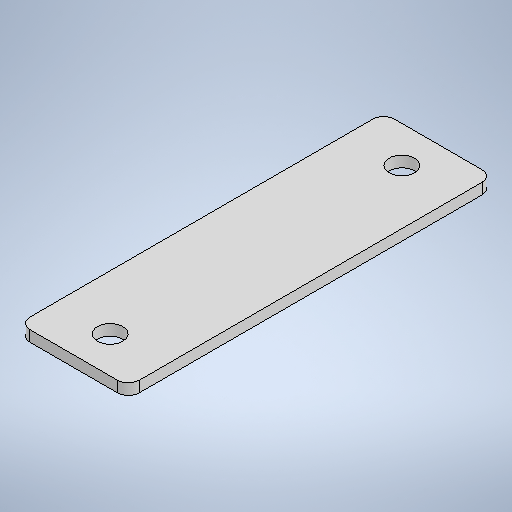
# Autodesk Inventor part: Part2
Saved by Autodesk Inventor 2025 (Build 290162010, 162A)
## iProperties
Created: 2025-11-03
Part Number: Part2
Material: Generic
Description: DIE16(5)|\ 90°|corrY -___°|X_____|bom___
Document SubType Name: Sheet Metal
Designer: admin
Stock Number: МОО 305 шпангоут борт
Mass: 186.989 g
Surface Area: 677.943 cm^2
Volume: 186.989 cm^3
Density: 1 g/cm^3
Sheet Metal Rule: Default
Sheet Metal Width: 0.000 mm
Sheet Metal Length: 0.000 mm
Sheet Metal Area: 0.000 mm^2
Appearance: Default
Author: admin
Autodesk Inventor part; units mm, degrees
ref_plane "YZ Plane" through (0, 0, 0) normal (1, 0, 0) x (0, 1, 0)
ref_plane "XZ Plane" through (0, 0, 0) normal (0, 1, 0) x (-1, 0, 0)
ref_plane "XY Plane" through (0, 0, 0) normal (0, 0, 1) x (1, 0, 0)
sketch "Sketch1" plane through (0, 0, 0) normal (0, 0, 1) x (1, 0, 0)
  line L0 (-30, -100) -> (30, -100)
  line L1 (30, -100) -> (30, 100)
  line L2 (30, 100) -> (-30, 100)
  line L3 (-30, 100) -> (-30, -100)
  line L4 (-30, -100) -> (30, 100) construction
  line L5 (30, -100) -> (-30, 100) construction
  circle A0 centre (0, 80) radius 7
  circle A1 centre (0, -80) radius 7
  line L6 (0, 100) -> (0, -100) construction
  line L7 (-30, 0) -> (30, 0) construction
  point P0 (0, 0)
  point P1 (0, 0)
  dimension "d154" = 60
  dimension "d155" = 200
  dimension "d157" = 20
  dimension "d159" = 14
  measures "d154" distance of L1.end L2.end
  measures "d155" distance of L0.end L1.end
  measures "d157" distance from line of L2 A0.centre
  measures "d159" diameter of A0
extrude "Plate5" add sketch "Sketch1" along normal blind 6
fillet "Corner Round1" radius 6 4 edges at (-30, 100, 3) (30, 100, 3) (30, -100, 3) (-30, -100, 3)
body "Solid3"
